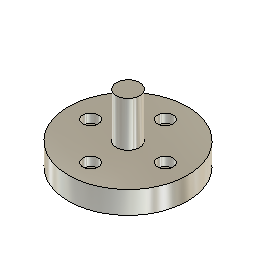
Top Cap For Metal Cylinder v1 (Autodesk Fusion 360 design; units mm, degrees)
Autodesk Fusion 360 part; units mm, degrees
cylinder "CylinderPrimitive1" add diameter 50.5 height 28.575 placed x (1, 0, 0) y (0, 1, 0) z (0, 0, 1) at (0, 0, 0)
sketch "Sketch2" plane through (0, 0, 28.575) normal (0, 0, 1) x (-1, 0, 0)
  circle A0 centre (0, 0) radius 25.25
  circle A1 centre (0, 0) radius 4.9
  dimension "d3" = 9.8
  constraint concentric A0 A1
  measures "d3" diameter of A1
extrude "Extrude1" cut sketch "Sketch2" against normal blind 19.05
sketch "Sketch3" plane through (0, 0, 9.525) normal (0, 0, 1) x (-1, 0, 0)
  circle A0 centre (0, 0) radius 4.9
  circle A1 centre (0, 0) radius 25.25
  line L0 (0, 0) -> (0, 15.875)
  line L1 (0, 0) -> (15.875, 0)
  line L2 (0, 0) -> (0, -15.875)
  line L3 (0, 0) -> (-15.875, 0)
  dimension "d6" = 15.875
  dimension "d7" = 15.875
  dimension "d8" = 15.875
  dimension "d9" = 15.875
  constraint coincident A0.centre A1.centre
  constraint vertical L0
  constraint horizontal L1
  constraint vertical L2
  constraint perpendicular L2 L3
  measures "d6" distance of A0.centre L0.end
  measures "d7" distance of A0.centre L1.end
  measures "d8" distance of A0.centre L2.end
  measures "d9" distance of A0.centre L3.end
hole "Hole1" at (-15.875, 0, 9.525) at (0, 15.875, 9.525) at (0, -15.875, 9.525) at (15.875, 0, 9.525) direction (0, 0, -1) diameter 3.9 depth 16.3 tip angle 180 counterbore diameter 6.6 counterbore depth 3.8
